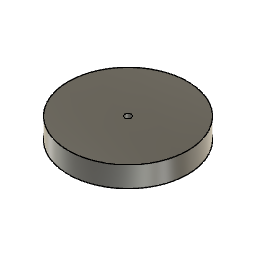
Robot Model (Autodesk Fusion 360 archive; units mm, degrees)
design "whl"
Autodesk Fusion 360 part; units mm, degrees
sketch "Sketch1" plane through (0, 0, 0) normal (0, 0, 1) x (1, 0, 0)
  circle A0 centre (0, 0) radius 3
  circle A1 centre (0, 0) radius 55
  dimension "d1" = 6
  dimension "d2" = 110
  constraint coincident A0.centre A1.centre
  constraint concentric A0 A1
  measures "d1" diameter of A0
  measures "d2" diameter of A1
extrude "Extrude1" add sketch "Sketch1" along normal mid plane 19

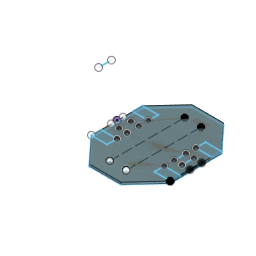
design "acrylic sheet v2"
Autodesk Fusion 360 part; units mm, degrees
sketch "Sketch1" plane through (0, 0, 0) normal (0, 0, 1) x (1, 0, 0)
  line L0 (0.4911, 119.2685) -> (0.4911, 249.2685)
  line L1 (200.4911, 249.2685) -> (200.4911, 119.2685)
  line L2 (60.4911, 314.2685) -> (140.4911, 314.2685)
  line L3 (140.4911, 314.2685) -> (200.4911, 249.2685)
  line L4 (60.4911, 314.2685) -> (0.4911, 249.2685)
  line L5 (60.4911, 54.2685) -> (140.4911, 54.2685)
  line L6 (200.4911, 119.2685) -> (140.4911, 54.2685)
  line L7 (0.4911, 119.2685) -> (60.4911, 54.2685)
  dimension "d2" = 130
  dimension "d11" = 80
  constraint vertical L0
  measures "d2" distance of L0.start L0.end
  measures "d11" distance of L2.start L2.end
extrude "Extrude1" add sketch "Sketch1" along normal blind 5
sketch "Sketch2" plane through (0, 0, 5) normal (0, 0, 1) x (-1, 0, 0)
  line L0 (-60.4911, -314.2685) -> (-0.4911, -249.2685)
  line L1 (-0.4911, -249.2685) -> (-0.4911, -119.2685)
  line L2 (-0.4911, -119.2685) -> (-60.4911, -54.2685)
  line L3 (-60.4911, -54.2685) -> (-140.4911, -54.2685)
  line L4 (-140.4911, -54.2685) -> (-200.4911, -119.2685)
  line L5 (-200.4911, -119.2685) -> (-200.4911, -249.2685)
  line L6 (-200.4911, -249.2685) -> (-140.4911, -314.2685)
  line L7 (-140.4911, -314.2685) -> (-60.4911, -314.2685)
  circle A0 centre (-79.7411, -86.7685) radius 1.5
  circle A1 centre (-121.2411, -86.7685) radius 1.5
  dimension "d19" = 3
  dimension "d22" = 3
  measures "d19" diameter of A0
  measures "d22" diameter of A1
hole "Hole1" at (79.7411, 86.7685, 5) direction (0, 0, -1) diameter 3 depth 5 tip angle 118
sketch "Sketch3" plane through (0, 0, 5) normal (0, 0, 1) x (-1, 0, 0)
  circle A0 centre (-79.7411, -86.7685) radius 1.5
  line L0 (-60.4911, -314.2685) -> (-0.4911, -249.2685)
  line L1 (-0.4911, -249.2685) -> (-0.4911, -119.2685)
  line L2 (-0.4911, -119.2685) -> (-60.4911, -54.2685)
  line L3 (-60.4911, -54.2685) -> (-140.4911, -54.2685)
  line L4 (-140.4911, -54.2685) -> (-200.4911, -119.2685)
  line L5 (-200.4911, -119.2685) -> (-200.4911, -249.2685)
  line L6 (-200.4911, -249.2685) -> (-140.4911, -314.2685)
  line L7 (-140.4911, -314.2685) -> (-60.4911, -314.2685)
  circle A1 centre (-121.2411, -86.7685) radius 1.5
hole "Hole2" at (121.2411, 86.7685, 5) direction (0, 0, -1) diameter 3 depth 5 tip angle 118
sketch "Sketch4" plane through (0, 0, 0) normal (0, 0, 1) x (1, 0, 0)
  line L0 (-144.6108, 315.3012) -> (-144.6108, 282.8012)
  dimension "d32" = 32.5
  constraint vertical L0
  measures "d32" distance of L0.start L0.end
sketch "Sketch5" plane through (0, 0, 5) normal (0, 0, 1) x (-1, 0, 0)
  circle A0 centre (-121.2411, -86.7685) radius 1.5
  circle A1 centre (-79.7411, -86.7685) radius 1.5
  line L0 (-60.4911, -314.2685) -> (-0.4911, -249.2685)
  line L1 (-0.4911, -249.2685) -> (-0.4911, -119.2685)
  line L2 (-0.4911, -119.2685) -> (-60.4911, -54.2685)
  line L3 (-60.4911, -54.2685) -> (-140.4911, -54.2685)
  line L4 (-140.4911, -54.2685) -> (-200.4911, -119.2685)
  line L5 (-200.4911, -119.2685) -> (-200.4911, -249.2685)
  line L6 (-200.4911, -249.2685) -> (-140.4911, -314.2685)
  line L7 (-140.4911, -314.2685) -> (-60.4911, -314.2685)
  line L8 (-79.7411, -86.7685) -> (-79.7411, -276.7685) construction
  line L9 (-121.2411, -86.7685) -> (-121.2411, -276.7685) construction
  circle A2 centre (-79.7411, -276.7685) radius 1.5
  circle A3 centre (-121.2411, -276.7685) radius 1.5
  dimension "d33" = 190
  dimension "d34" = 190
  dimension "d35" = 3
  dimension "d36" = 3
  constraint coincident A1.centre L8.start
  constraint vertical L8
  constraint coincident A0.centre L9.start
  constraint vertical L9
  constraint coincident L8.end A2.centre
  constraint coincident L9.end A3.centre
  measures "d33" distance of A1.centre L8.end
  measures "d34" distance of A0.centre L9.end
  measures "d35" diameter of A2
  measures "d36" diameter of A3
extrude "Extrude2" cut sketch "Sketch5" along normal mid plane 10 contours A2
extrude "Extrude3" cut sketch "Sketch5" along normal mid plane 12 contours A3
sketch "Sketch6" plane through (0, 0, 5) normal (0, 0, 1) x (-1, 0, 0)
  line L0 (0, -120) -> (0, -185) construction
  dimension "d41" = 65
  constraint vertical L0
  measures "d41" distance of L0.start L0.end
sketch "Sketch7" plane through (0, 0, 5) normal (0, 0, 1) x (-1, 0, 0)
  line L0 (-20, -170) -> (-18.5, -170)
  line L1 (0, -170) -> (0, -200)
  line L2 (-18.5, -200) -> (-20, -200)
  line L3 (-200.4911, -119.2685) -> (-200.4911, -184.2685)
  line L4 (-181.9911, -169.2685) -> (-180.4911, -169.2685)
  line L5 (-180.4911, -169.2685) -> (-180.4911, -199.2685)
  line L6 (-180.4911, -199.2685) -> (-181.9911, -199.2685)
  line L7 (-200.4911, -199.2685) -> (-200.4911, -169.2685)
  line L8 (-160.4911, -169.2685) -> (-160.4911, -199.2685)
  circle A0 centre (-180.4911, -169.2685) radius 1.5
  circle A1 centre (-160.4911, -169.2685) radius 1.5
  circle A2 centre (-180.4911, -199.2685) radius 1.5
  circle A3 centre (-160.4911, -199.2685) radius 1.5
  circle A4 centre (-40, -170) radius 1.5
  circle A5 centre (-40, -200) radius 1.5
  circle A6 centre (-20, -170) radius 1.5
  circle A7 centre (-20, -200) radius 1.5
  line L9 (-20, -170) -> (-21.5, -170)
  line L10 (-38.5, -170) -> (-40, -170)
  line L11 (-20, -200) -> (-20, -198.5)
  line L12 (-20, -171.5) -> (-20, -170)
  line L13 (-40, -170) -> (-40, -171.5)
  line L14 (-40, -198.5) -> (-40, -200)
  line L15 (-40, -200) -> (-38.5, -200)
  line L16 (-21.5, -200) -> (-20, -200)
  line L17 (-20, -200) -> (-20, -198.5)
  line L18 (-20, -171.5) -> (-20, -170)
  line L19 (-160.4911, -199.2685) -> (-161.9911, -199.2685)
  line L20 (-178.9911, -199.2685) -> (-180.4911, -199.2685)
  line L21 (-180.4911, -169.2685) -> (-178.9911, -169.2685)
  line L22 (-161.9911, -169.2685) -> (-160.4911, -169.2685)
  line L23 (-180.4911, -199.2685) -> (-180.4911, -197.7685)
  line L24 (-180.4911, -170.7685) -> (-180.4911, -169.2685)
  point P0 (0, -185)
  point P1 (-200.4911, -119.2685)
  dimension "d42" = 20
  dimension "d43" = 30
  dimension "d44" = 65
  dimension "d45" = 20
  dimension "d46" = 30
  dimension "d47" = 20
  dimension "d48" = 30
  dimension "d49" = 30
  dimension "d50" = 3
  dimension "d51" = 3
  dimension "d52" = 3
  dimension "d53" = 3
  dimension "d54" = 3
  dimension "d55" = 3
  dimension "d56" = 3
  dimension "d57" = 3
  constraint horizontal L0
  constraint vertical L1
  constraint horizontal L2
  constraint vertical L17
  constraint midpoint L1 P0
  constraint vertical L3
  constraint horizontal L4
  constraint vertical L5
  constraint horizontal L6
  constraint vertical L7
  constraint midpoint L3.end L7
  constraint coincident P1 L3.start
  constraint horizontal L21
  constraint vertical L8
  constraint horizontal L19
  constraint vertical L23
  constraint horizontal L9
  constraint vertical L13
  constraint horizontal L15
  constraint vertical L11
  constraint coincident L4.end L5.start
  constraint coincident L8.start A1.centre
  constraint coincident L5.end L6.start
  constraint coincident L8.end A3.centre
  constraint coincident A4.centre L10.end
  constraint coincident A5.centre L14.end
  constraint coincident L0.start A6.centre
  constraint coincident L2.end A7.centre
  constraint coincident A6 L9.end
  constraint coincident A4 L10.start
  constraint collinear L9 L10
  constraint coincident A6 L0.end
  constraint coincident A7 L11.end
  constraint coincident A6 L12.start
  constraint collinear L11 L12
  constraint coincident A4 L13.end
  constraint coincident A5 L14.start
  constraint collinear L13 L14
  constraint coincident A5 L15.end
  constraint coincident A7 L16.start
  constraint collinear L15 L16
  constraint collinear L17 L18
  constraint coincident A7 L2.start
  constraint coincident A2 L6.end
  constraint coincident A3 L19.end
  constraint coincident A2 L20.start
  constraint collinear L19 L20
  constraint coincident A0 L21.end
  constraint coincident A1 L22.start
  constraint collinear L21 L22
  constraint coincident A0 L4.start
  constraint coincident A2 L23.end
  constraint coincident A0 L24.start
  constraint collinear L23 L24
  measures "d42" distance of L0.start L1.start
  measures "d43" distance of L0.start L2.end
  measures "d44" distance of P1 L3.end
  measures "d45" distance of L7.end L4.end
  measures "d46" distance of L7.end L7.start
  measures "d47" distance of L4.end L8.start
  measures "d48" distance of L4.end L5.end
  measures "d49" distance of L0.start L2.end
  measures "d50" diameter of A0
  measures "d51" diameter of A1
  measures "d52" diameter of A2
  measures "d53" diameter of A3
  measures "d54" diameter of A4
  measures "d55" diameter of A5
  measures "d56" diameter of A6
  measures "d57" diameter of A7
extrude "Extrude4" cut sketch "Sketch7" along normal mid plane 10 contours L0 A6 L9 | A6 L9 L12 L18 | L0 A6 L12 L18 | L2 A7 L16 | L2 A7 L11 L17 | A7 L11 L16 L17 | A4 L10 L13 | A4 L10 L13 | A5 L14 L15 | A5 L14 L15
extrude "Extrude5" cut sketch "Sketch7" along normal mid plane 10 contours L8 A1 L22 | L8 A1 L22
extrude "Extrude6" cut sketch "Sketch7" along normal mid plane 10 contours L4 A0 L21 | L4 L5 A0 L24 | L5 A0 L21 L24
sketch "Sketch8" plane through (0, 0, 5) normal (0, 0, 1) x (-1, 0, 0)
extrude "Extrude7" cut sketch "Sketch7" along normal mid plane 10 contours L8 A3 L19 | L8 A3 L19
extrude "Extrude8" cut sketch "Sketch7" along normal mid plane 10 contours L5 L6 A2 L23
extrude "Extrude9" cut sketch "Sketch7" along normal mid plane 10 contours L5 A2 L20 L23
extrude "Extrude10" cut sketch "Sketch7" along normal mid plane 10 contours L6 A2 L20
sketch "Sketch9" plane through (0, 0, 5) normal (0, 0, 1) x (-1, 0, 0)
  line L0 (-200.4912, -249.2683) -> (-160.4912, -249.2683)
  line L1 (-160.4912, -249.2683) -> (-160.4912, -224.2683)
  line L2 (-160.4912, -224.2683) -> (-200.4912, -224.2683)
  line L3 (-200.4912, -224.2683) -> (-200.4912, -249.2683)
  line L4 (-200.4912, -119.2686) -> (-160.4912, -119.2686)
  line L5 (-160.4912, -119.2686) -> (-160.4912, -144.2686)
  line L6 (-160.4912, -144.2686) -> (-200.4912, -144.2686)
  line L7 (-200.4912, -144.2686) -> (-200.4912, -119.2686)
  line L8 (-0.4911, -119.2687) -> (-40.4911, -119.2687)
  line L9 (-40.4911, -119.2687) -> (-40.4911, -144.2687)
  line L10 (-40.4911, -144.2687) -> (-0.4911, -144.2687)
  line L11 (-0.4911, -144.2687) -> (-0.4911, -119.2687)
  line L12 (-0.4911, -249.2686) -> (-40.4911, -249.2686)
  line L13 (-40.4911, -249.2686) -> (-40.4911, -224.2686)
  line L14 (-40.4911, -224.2686) -> (-0.4911, -224.2686)
  line L15 (-0.4911, -224.2686) -> (-0.4911, -249.2686)
  circle A0 centre (-40.4911, -144.2687) radius 1.5
  circle A1 centre (-160.4912, -144.2686) radius 1.5
  circle A2 centre (-40.4911, -224.2686) radius 1.5
  circle A3 centre (-160.4912, -224.2683) radius 1.5
  dimension "d72" = 40
  dimension "d73" = 25
  dimension "d74" = 40
  dimension "d75" = 25
  dimension "d76" = 40
  dimension "d77" = 25
  dimension "d78" = 40
  dimension "d79" = 25
  dimension "d80" = 3
  dimension "d81" = 3
  dimension "d82" = 3
  dimension "d83" = 3
  constraint horizontal L0
  constraint vertical L1
  constraint horizontal L2
  constraint vertical L3
  constraint horizontal L4
  constraint vertical L5
  constraint horizontal L6
  constraint vertical L7
  constraint horizontal L8
  constraint vertical L9
  constraint horizontal L10
  constraint vertical L11
  constraint horizontal L12
  constraint vertical L13
  constraint horizontal L14
  constraint vertical L15
  constraint coincident L9.end L10.start
  constraint coincident L5.end L6.start
  constraint coincident L13.end L14.start
  constraint coincident L1.end L2.start
  measures "d72" distance of L0.start L0.end
  measures "d73" distance of L0.start L2.end
  measures "d74" distance of L4.start L4.end
  measures "d75" distance of L4.start L6.end
  measures "d76" distance of L8.start L8.end
  measures "d77" distance of L8.start L10.end
  measures "d78" distance of L12.start L12.end
  measures "d79" distance of L12.start L14.end
  measures "d80" diameter of A0
  measures "d81" diameter of A1
  measures "d82" diameter of A2
  measures "d83" diameter of A3
extrude "Extrude11" cut sketch "Sketch9" along normal mid plane 10 contours L9 L10 A0 picked at (-41.438, -143.9558)
extrude "Extrude12" cut sketch "Sketch9" along normal mid plane 10 contours L9 L10 A0 picked at (-39.8933, -143.4702)
extrude "Extrude13" cut sketch "Sketch9" along normal mid plane 10 contours L13 L14 A2 | L13 L14 A2
extrude "Extrude14" cut sketch "Sketch9" along normal mid plane 10 contours L1 L2 A3 picked at (-161.1695, -223.5373)
extrude "Extrude15" cut sketch "Sketch9" along normal mid plane 10 contours L1 L2 A3 picked at (-161.4861, -224.3395)
extrude "Extrude16" cut sketch "Sketch9" along normal mid plane 10 contours L5 L6 A1 picked at (-161.4856, -144.3432)
extrude "Extrude17" cut sketch "Sketch9" along normal mid plane 10 contours L5 L6 A1 picked at (-161.1965, -143.5633)

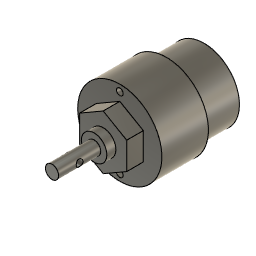
design "HW-DC MOTOR v1"
Autodesk Fusion 360 part; units mm, degrees
sketch "Sketch1" plane through (0, 0, 0) normal (0, 1, 0) x (1, 0, 0)
  circle A0 centre (0, 0) radius 19
  dimension "d1" = 38
  constraint coincident A0.centre origin
  measures "d1" diameter of A0
extrude "Extrude1" add sketch "Sketch1" along normal blind 21
sketch "Sketch2" plane through (0, 21, 0) normal (0, 1, 0) x (-1, 0, 0)
  circle A0 centre (0, 0) radius 19
  circle A1 centre (0, 0) radius 16
  dimension "d4" = 32
  constraint concentric A0 A1
  measures "d4" diameter of A1
extrude "Extrude2" add sketch "Sketch2" along normal blind 17 contours A1
sketch "Sketch3" plane through (0, 0, 0) normal (0, 1, 0) x (1, 0, 0)
  line L0 (0, -12.25) -> (10.6088, -6.125)
  line L1 (10.6088, -6.125) -> (10.6088, 6.125)
  line L2 (10.6088, 6.125) -> (0, 12.25)
  line L3 (0, 12.25) -> (-10.6088, 6.125)
  line L4 (-10.6088, 6.125) -> (-10.6088, -6.125)
  line L5 (-10.6088, -6.125) -> (0, -12.25)
  dimension "d7" = 12.25
  measures "d7" distance of L0.start origin
sketch "Sketch4" plane through (0, 0, 0) normal (0, 1, 0) x (1, 0, 0)
extrude "Extrude3" add sketch "Sketch3" against normal blind 7.5
sketch "Sketch5" plane through (0, 0, 0) normal (0, 1, 0) x (1, 0, 0)
sketch "Sketch6" plane through (0, -7.5, 0) normal (0, -1, 0) x (1, 0, 0)
  line L0 (0, 12.25) -> (-10.6088, 6.125)
  line L1 (-10.6088, 6.125) -> (-10.6088, -6.125)
  line L2 (-10.6088, -6.125) -> (0, -12.25)
  line L3 (0, -12.25) -> (10.6088, -6.125)
  line L4 (10.6088, -6.125) -> (10.6088, 6.125)
  line L5 (10.6088, 6.125) -> (0, 12.25)
  circle A0 centre (0, 0) radius 5.75
  dimension "d10" = 11.5
  constraint coincident A0.centre origin
  measures "d10" diameter of A0
extrude "Extrude4" add sketch "Sketch6" along normal blind 4.1 contours A0
sketch "Sketch7" plane through (0, -11.6, 0) normal (0, -1, 0) x (1, 0, 0)
  circle A0 centre (0, 0) radius 5.75
  circle A1 centre (0, 0) radius 3
  dimension "d13" = 6
  constraint concentric A0 A1
  measures "d13" diameter of A1
extrude "Extrude5" add sketch "Sketch7" along normal blind 19 contours A1
sketch "Sketch8" plane through (0, 0, 0) normal (1, 0, 0) x (0, 1, 0)
  circle A0 centre (-21.1, 0) radius 1.55
  point P0 (-30.6, 0)
  dimension "d16" = 3.1
  dimension "d17" = 9.5
  measures "d16" diameter of A0
  measures "d17" distance of A0.centre P0
extrude "Extrude6" cut sketch "Sketch8" along normal through all and the other way through all
sketch "Sketch9" plane through (0, 0, 0) normal (0, 1, 0) x (1, 0, 0)
  circle A0 centre (-15, 0) radius 1.5
  dimension "d20" = 3
  measures "d20" diameter of A0
extrude "Extrude7" cut sketch "Sketch9" along normal blind 21
mirror "Mirror1" about plane through (0, 0, 0) normal (1, 0, 0) of "Extrude7"
extrude "Extrude8" add sketch "Sketch9" along normal blind 21
extrude "Extrude9" add sketch "Sketch1" along normal blind 21
sketch "Sketch10" plane through (0, 0, 0) normal (0, 1, 0) x (1, 0, 0)
  line L0 (0, 0) -> (0, -16)
  line L1 (0, 0) -> (0, 16)
  circle A0 centre (0, -16) radius 1.5
  circle A1 centre (0, 16) radius 1.5
  dimension "d29" = 16
  dimension "d30" = 16
  dimension "d31" = 3
  dimension "d32" = 3
  constraint coincident L0.start L1.start
  constraint vertical L0
  constraint parallel L0 L1
  constraint coincident L0.end A0.centre
  constraint coincident L1.end A1.centre
  measures "d29" distance of L0.start L0.end
  measures "d30" distance of L0.start L1.end
  measures "d31" diameter of A0
  measures "d32" diameter of A1
extrude "Extrude10" cut sketch "Sketch10" along normal blind 21

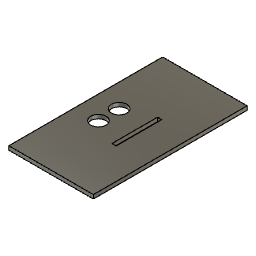
design "finalmouth"
Autodesk Fusion 360 part; units mm, degrees
sketch "Sketch1" plane through (0, 0, 0) normal (0, 0, 1) x (1, 0, 0)
  line L0 (0, 0) -> (110, 0)
  line L1 (110, 0) -> (110, 200)
  line L2 (110, 200) -> (0, 200)
  line L3 (0, 200) -> (0, 0)
  line L4 (30, 100) -> (30, 113.5)
  line L5 (30, 100) -> (30, 86.5)
  circle A0 centre (30, 113.5) radius 10
  circle A1 centre (30, 86.5) radius 10
  line L6 (64.5639, 69.7592) -> (70, 69.7592)
  line L7 (70, 69.7592) -> (70, 128.9006)
  line L8 (70, 128.9006) -> (64.5639, 128.9006)
  line L9 (64.5639, 128.9006) -> (64.5639, 69.7592)
  dimension "d1" = 110
  dimension "d2" = 200
  dimension "d3" = 13.5
  dimension "d4" = 13.5
  dimension "d5" = 20
  dimension "d6" = 20
  constraint horizontal L0
  constraint vertical L1
  constraint horizontal L2
  constraint vertical L3
  constraint coincident L0.start L3.end
  constraint parallel L3 L4
  constraint parallel L4 L5
  constraint coincident L4.end A0.centre
  constraint coincident L5.end A1.centre
  constraint horizontal L6
  constraint vertical L7
  constraint horizontal L8
  constraint vertical L9
  measures "d1" distance of L0.start L0.end
  measures "d2" distance of L0.start L2.end
  measures "d3" distance of L4.start L4.end
  measures "d4" distance of L4.start L5.end
  measures "d5" diameter of A0
  measures "d6" diameter of A1
extrude "Extrude1" add sketch "Sketch1" along normal blind 5

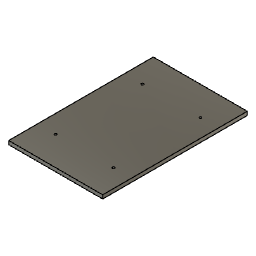
design "base130_200"
Autodesk Fusion 360 part; units mm, degrees
sketch "Sketch1" plane through (0, 0, 0) normal (0, 0, 1) x (1, 0, 0)
  line L0 (0, 0) -> (130, 0)
  line L1 (130, 0) -> (130, 200)
  line L2 (130, 200) -> (0, 200)
  line L3 (0, 200) -> (0, 0)
  circle A0 centre (25, 160) radius 1.5
  circle A1 centre (105, 160) radius 1.5
  circle A2 centre (25, 40) radius 1.5
  circle A3 centre (105, 40) radius 1.5
  dimension "d1" = 130
  dimension "d2" = 200
  dimension "d11" = 3
  dimension "d12" = 3
  dimension "d13" = 3
  dimension "d14" = 3
  constraint horizontal L0
  constraint vertical L1
  constraint horizontal L2
  constraint vertical L3
  constraint coincident L0.start L3.end
  measures "d1" distance of L0.start L0.end
  measures "d2" distance of L0.start L2.end
  measures "d11" diameter of A0
  measures "d12" diameter of A1
  measures "d13" diameter of A2
  measures "d14" diameter of A3
extrude "Extrude1" add sketch "Sketch1" along normal blind 5

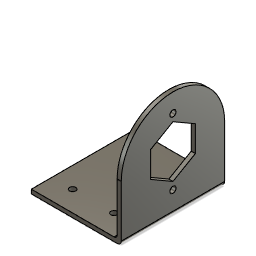
design "motor_mount 123"
Autodesk Fusion 360 part; units mm, degrees
sketch "Sketch1" plane through (0, 0, 0) normal (1, 0, 0) x (0, 0, -1)
  line L0 (0, 0) -> (-30, 0)
  line L1 (-30, 0) -> (30, 0)
  line L2 (30, 0) -> (30, 30)
  line L3 (-30, 30) -> (-30, 0)
  line L4 (0, 0) -> (0, 30)
  circle A0 centre (0, 30) radius 13.25
  arc A1 (30, 30) -> (-30, 30) centre (0, 30) ccw
  circle A2 centre (0, 30) radius 17.5
  line L5 (0, 30) -> (17.5, 30) construction
  circle A3 centre (-12.3744, 42.3744) radius 2.1
  circle A4 centre (12.3744, 42.3744) radius 2.1
  circle A5 centre (-12.3744, 17.6256) radius 2.1
  circle A6 centre (12.3744, 17.6256) radius 2.1
  dimension "d1" = 30
  dimension "d2" = 60
  dimension "d8" = 4.2
  dimension "d9" = 4.2
  dimension "d10" = 4.2
  dimension "d11" = 4.2
  constraint horizontal L0
  constraint horizontal L1
  constraint vertical L2
  constraint vertical L3
  constraint perpendicular L0 L4
  constraint coincident L4.end A0.centre
  constraint concentric A0 A1
  constraint concentric A1 A2
  constraint horizontal L5
  measures "d1" distance of L0.start L0.end
  measures "d2" distance of L0.end L1.end
  measures "d8" diameter of A3
  measures "d9" diameter of A4
  measures "d10" diameter of A5
  measures "d11" diameter of A6
extrude "Extrude1" add sketch "Sketch1" along normal blind 2 contours L0 L1 L2 L3 A1 | A2 A3 A4 A5 A6
sketch "Sketch2" plane through (0, 0, 0) normal (-1, 0, 0) x (0, 0, 1)
  circle A0 centre (12.3744, 42.3744) radius 2.1
  circle A1 centre (-12.3744, 42.3744) radius 2.1
  circle A2 centre (-12.3744, 17.6256) radius 2.1
  circle A3 centre (0, 30) radius 13.25
  circle A4 centre (12.3744, 17.6256) radius 2.1
  arc A5 (30, 30) -> (-30, 30) centre (0, 30) ccw
  line L0 (-30, 30) -> (-30, 0)
  line L1 (-30, 0) -> (30, 0)
  line L2 (30, 0) -> (30, 30)
  line L3 (-30, 0) -> (30, 0)
  line L4 (30, 0) -> (30, 2)
  line L5 (30, 2) -> (-30, 2)
  line L6 (-30, 2) -> (-30, 0)
  dimension "d14" = 2
  constraint horizontal L3
  constraint vertical L4
  constraint horizontal L5
  constraint vertical L6
  constraint coincident L0.end L1.start
  measures "d14" distance of L0.end L5.end
extrude "Extrude2" add sketch "Sketch2" along normal blind 61.93 contours L0 L1 L2 L3 L4 L5 L6
fillet "Fillet1" radius 2 1 edges at (2, 0, 0)
fillet "Fillet2" radius 1.5 1 edges at (0, 2, 0)
sketch "Sketch3" plane through (0, 2, 0) normal (0, 1, 0) x (-1, 0, 0)
  line L0 (1.5, 30) -> (1.5, -30)
  line L1 (1.5, -30) -> (61.93, -30)
  line L2 (61.93, -30) -> (61.93, 30)
  line L3 (61.93, 30) -> (1.5, 30)
  line L4 (61.93, 30) -> (61.93, 23)
  circle A0 centre (55.6, 23) radius 2.15
  line L5 (61.93, -30) -> (61.93, -23)
  line L6 (61.93, -23) -> (55.6, -23)
  circle A1 centre (55.6, -23) radius 2.15
  line L7 (-2, -30) -> (12, -30)
  line L8 (12, -30) -> (12, -23)
  circle A2 centre (12, -23) radius 2.15
  line L9 (12, -23) -> (12, 23)
  circle A3 centre (12, 23) radius 2.15
  line L10 (12, 23) -> (55.6, 23)
  point P0 (-2, -30)
  dimension "d22" = 6.33
  dimension "d23" = 4.3
  dimension "d24" = 7
  dimension "d25" = 6.33
  dimension "d26" = 4.3
  dimension "d27" = 14
  dimension "d28" = 7
  dimension "d29" = 4.3
  dimension "d30" = 46
  dimension "d31" = 4.3
  constraint coincident L2.end L3.start
  constraint perpendicular L3 L4
  constraint coincident L1.end L2.start
  constraint perpendicular L1 L5
  constraint perpendicular L2 L6
  constraint coincident L6.end A1.centre
  constraint coincident P0 L7.start
  constraint perpendicular L0 L7
  constraint perpendicular L1 L8
  constraint coincident L8.end A2.centre
  constraint perpendicular L1 L9
  constraint coincident L9.end A3.centre
  constraint coincident A0.centre L10.end
  measures "d22" distance of L4.end A0.centre
  measures "d23" diameter of A0
  measures "d24" distance of L1.end L5.end
  measures "d25" distance of L5.end L6.end
  measures "d26" diameter of A1
  measures "d27" distance of P0 L7.end
  measures "d28" distance of L7.end L8.end
  measures "d29" diameter of A2
  measures "d30" distance of L8.end L9.end
  measures "d31" diameter of A3
extrude "Extrude3" cut sketch "Sketch3" against normal through all contours A0 | A1 | L8 A2 L9 | L8 A2 L9 | L9 A3 L10 | L9 A3 L10
sketch "Sketch4" plane through (2, 0, 0) normal (1, 0, 0) x (0, 0, -1)
  line L0 (-30, 2) -> (30, 2)
  line L1 (30, 2) -> (30, 30)
  arc A0 (30, 30) -> (-30, 30) centre (0, 30) ccw
  line L2 (-30, 30) -> (-30, 2)
  circle A1 centre (-12.3744, 17.6256) radius 2.1
  circle A2 centre (0, 30) radius 13.25
  circle A3 centre (12.3744, 17.6256) radius 2.1
  circle A4 centre (12.3744, 42.3744) radius 2.1
  circle A5 centre (-12.3744, 42.3744) radius 2.1
extrude "Extrude4" add sketch "Sketch4" against normal blind 2 contours A1 | A2 | A3 | A4 | A5
sketch "Sketch5" plane through (2, 0, 0) normal (1, 0, 0) x (0, 0, -1)
  line L0 (-30, 2) -> (30, 2)
  line L1 (30, 2) -> (30, 30)
  arc A0 (30, 30) -> (-30, 30) centre (0, 30) ccw
  line L2 (-30, 30) -> (-30, 2)
  line L3 (-30, 2) -> (20, 2)
  line L4 (20, 2) -> (20, 27)
  line L5 (20, 27) -> (-30, 27)
  line L6 (-30, 27) -> (-30, 2)
  arc A1 (20, 27) -> (-30, 27) centre (-5, 27) ccw
  dimension "d35" = 50
  dimension "d36" = 25
  dimension "d37" = 50
  constraint horizontal L3
  constraint vertical L4
  constraint horizontal L5
  constraint vertical L6
  constraint coincident L0.start L2.end
  constraint midpoint L5 A1.centre
  measures "d35" distance of L0.start L3.end
  measures "d36" distance of L0.start L5.end
  measures "d37" diameter of A1
extrude "Extrude5" cut sketch "Sketch5" against normal blind 2 contours L0 L1 A0 L2 L4 A1
sketch "Sketch6" plane through (2, 0, 0) normal (1, 0, 0) x (0, 0, -1)
  arc A0 (20, 27) -> (-30, 27) centre (-5, 27) ccw
  line L0 (-30, 27) -> (-30, 2)
  line L1 (-30, 2) -> (20, 2)
  line L2 (20, 2) -> (20, 27)
  line L3 (20, 2) -> (30, 2)
  line L4 (30, 2) -> (30, 0)
  line L5 (30, 0) -> (20, 0)
  line L6 (20, 0) -> (20, 2)
  dimension "d40" = 10
  dimension "d41" = 2
  constraint horizontal L3
  constraint vertical L4
  constraint horizontal L5
  constraint vertical L6
  constraint coincident L1.end L2.start
  measures "d40" distance of L1.end L3.end
  measures "d41" distance of L1.end L5.end
extrude "Extrude6" cut sketch "Sketch6" against normal blind 65 contours L3 L4 L5 L6
extrude "Extrude7" cut 1 faces at (0, 2.5, -26.6667) along direction (-1, 0, 0) blind 2
sketch "Sketch7" plane through (2, 0, 0) normal (1, 0, 0) x (0, 0, -1)
  arc A0 (20, 27) -> (-30, 27) centre (-5, 27) ccw
  line L0 (-30, 27) -> (-30, 2)
  line L1 (-30, 2) -> (20, 2)
  line L2 (20, 2) -> (20, 27)
  line L3 (20, 27) -> (-30, 27) construction
  line L4 (5.8253, 33.25) -> (-5, 39.5)
  line L5 (-5, 39.5) -> (-15.8253, 33.25)
  line L6 (-15.8253, 33.25) -> (-15.8253, 20.75)
  line L7 (-15.8253, 20.75) -> (-5, 14.5)
  line L8 (-5, 14.5) -> (5.8253, 20.75)
  line L9 (5.8253, 20.75) -> (5.8253, 33.25)
  circle A1 centre (-5, 43) radius 1.5
  circle A2 centre (-5, 11) radius 1.5
  point P0 (-5, 27)
  dimension "d46" = 12.5
  dimension "d47" = 3
  dimension "d48" = 3
  dimension "d49" = 16
  dimension "d50" = 32
  constraint coincident A0.start L2.end
  constraint coincident A0.end L0.start
  constraint coincident P0 A0.centre
  constraint collinear L4.end P0 A1.centre
  constraint collinear P0 A1.centre A2.centre
  constraint perpendicular L3 L9
  measures "d46" distance of L4.start P0
  measures "d48" diameter of A2
  measures "d49" vertical distance of P0 A1.centre
  measures "d50" vertical distance of A1.centre A2.centre
extrude "Extrude8" cut sketch "Sketch7" against normal blind 2 contours L4 L5 L6 L7 L8 L9 | A1 | A2
sketch "Sketch8" plane through (0, 2, 0) normal (0, 1, 0) x (-1, 0, 0)
  line L0 (1.5, -20) -> (61.93, -20)
  line L1 (61.93, -20) -> (61.93, 30)
  line L2 (61.93, 30) -> (1.5, 30)
  line L3 (1.5, 30) -> (1.5, -20)
  circle A0 centre (55.6, 23) radius 2.15
  circle A1 centre (12, 23) radius 2.15
  line L4 (1.5, -20) -> (41.5, -20)
  line L5 (41.5, -20) -> (41.5, 30)
  line L6 (41.5, 30) -> (1.5, 30)
  line L7 (1.5, 30) -> (1.5, -20)
  dimension "d53" = 40
  constraint horizontal L4
  constraint vertical L5
  constraint horizontal L6
  constraint vertical L7
  constraint coincident L0.start L3.end
  measures "d53" distance of L0.start L4.end
extrude "Extrude9" cut sketch "Sketch8" against normal blind 2 contours L0 L1 L2 L5
sketch "Sketch9" plane through (0, 0, 0) normal (0, 1, 0) x (1, 0, 0)
extrude "Extrude10" add sketch "Sketch8" sketch "Sketch3" against normal blind 2 contours A1 of sketch 2 contours L9 A3 L10 picked at (11.8948, 21.5744)
sketch "Sketch10" plane through (0, 0, 0) normal (0, 1, 0) x (1, 0, 0)
  circle A0 centre (-31.5, 10) radius 1.5
  circle A1 centre (-11.5, 10) radius 1.5
  circle A2 centre (-11.5, -20) radius 1.5
  circle A3 centre (-31.5, -20) radius 1.5
  line L0 (-1.5, 20) -> (-41.5, 20)
  line L1 (-41.5, -30) -> (-1.5, -30)
  line L2 (-41.5, 20) -> (-41.5, -30)
  line L3 (-1.5, -30) -> (-1.5, 20)
  dimension "d58" = 3
  dimension "d59" = 3
  dimension "d60" = 3
  dimension "d61" = 3
  dimension "d62" = 10
  dimension "d63" = 10
  dimension "d64" = 10
  dimension "d65" = 10
  dimension "d66" = 10
  dimension "d67" = 10
  dimension "d68" = 10
  dimension "d69" = 10
  measures "d58" diameter of A0
  measures "d59" diameter of A1
  measures "d60" diameter of A2
  measures "d61" diameter of A3
  measures "d62" distance of A1.centre L0
  measures "d63" distance of A2.centre L1
  measures "d64" distance of A0.centre L0
  measures "d65" distance of A3.centre L1
  measures "d66" distance of A3.centre L2
  measures "d67" distance of A0.centre L2
  measures "d68" distance of A1.centre L3
  measures "d69" distance of A2.centre L3
extrude "Extrude11" cut sketch "Sketch10" along normal blind 2 contours A0 | A1 | A2 | A3
